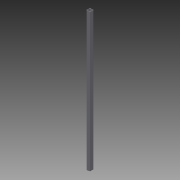
# Autodesk Inventor part: Square Tube 4
Saved by Autodesk Inventor 2013 (Build 170138000, 138)
## iProperties
Created: 2013-01-24
Part Number: Square Tube 4
Material: Generic
Document SubType Name: Modeling
Designer: actoennies
Density: 1 g/cm^3
Author: actoennies
Autodesk Inventor part; units mm, degrees
ref_plane "YZ Plane" through (0, 0, 0) normal (1, 0, 0) x (0, 1, 0)
ref_plane "XZ Plane" through (0, 0, 0) normal (0, 1, 0) x (-1, 0, 0)
ref_plane "XY Plane" through (0, 0, 0) normal (0, 0, 1) x (1, 0, 0)
sketch "Sketch1" plane through (0, 0, 0) normal (0, 1, 0) x (-1, 0, 0)
  line L0 (0, 0) -> (-25.4, 0)
  line L1 (-25.4, 0) -> (-25.4, 25.4)
  line L2 (-25.4, 25.4) -> (0, 25.4)
  line L3 (0, 25.4) -> (0, 0)
  line L4 (-1.5875, 23.8125) -> (-23.8125, 23.8125)
  line L5 (-23.8125, 23.8125) -> (-23.8125, 1.5875)
  line L6 (-23.8125, 1.5875) -> (-1.5875, 1.5875)
  line L7 (-1.5875, 1.5875) -> (-1.5875, 23.8125)
  dimension "d0" = 25.4
  dimension "d2" = 25.4
  dimension "d3" = 1.5875
  constraints: 16 end point, 4 parallel, 2 perpendicular, 1 horizontal, 3 other
  measures "d0" distance of L1.end L2.end
  measures "d2" distance of L0.end L1.end
  measures "d3" distance between parallel lines of L2 L4
extrude "Extrusion1" add sketch "Sketch1" along normal blind 1016
ref_plane "Work Plane1" through (102.0769, 3.5287, 0.7496) normal (0.0123379, -0.1467937, -0.9890902) x (-0.157097, 0.9765967, -0.1468992)
sketch "Sketch4" plane through (102.0769, 3.5287, 0.7496) normal (0.0123379, -0.1467937, -0.9890902) x (-0.157097, 0.9765967, -0.1468992)
  line L0 (12.7, -101.348) -> (12.7, -75.0726)
  line L1 (12.7, -75.0726) -> (-1.1984, -75.0726)
  line L2 (-1.1984, -75.0726) -> (-1.1984, -113.5605)
  line L3 (-1.1984, -113.5605) -> (12.7, -101.348)
  constraints: 8 end point, 2 perpendicular, 1 vertical
extrude "Extrusion3" cut sketch "Sketch4" along normal mid plane 2540
ref_plane "Work Plane2" through (2.7066, 641.7405, 200.1131) normal (-0.157097, 0.9765967, -0.1468992) x (0.9875061, 0.1571955, -0.0110117)
sketch "Sketch5" plane through (2.7066, 641.7405, 200.1131) normal (-0.157097, 0.9765967, -0.1468992) x (0.9875061, 0.1571955, -0.0110117)
  line L0 (-64.0002, -43.7034) -> (-64.0002, 400.9318)
  line L1 (-64.0002, 400.9318) -> (260.4368, 400.9318)
  line L2 (260.4368, 400.9318) -> (260.4368, -43.7034)
  line L3 (260.4368, -43.7034) -> (-64.0002, -43.7034)
  point P0 (-101.348, 292.1)
  constraints: 8 end point, 2 parallel, 1 perpendicular, 1 vertical
extrude "Extrusion4" cut sketch "Sketch5" along normal blind 2540
body "Solid1"
